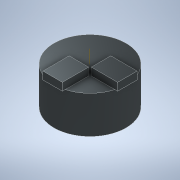
# Autodesk Inventor part: top tvc
Saved by Autodesk Inventor 2021 (Build 250183000, 183)
## iProperties
Created: 2021-07-19
Part Number: top tvc
Material: Iron, Cast
Document SubType Name: Modeling
Designer: samlo
Density: 7.15 g/cm^3
Appearance: Iron Gray
Author: samlo
Autodesk Inventor part; units mm, degrees
ref_plane "YZ Plane" through (0, 0, 0) normal (1, 0, 0) x (0, 1, 0)
ref_plane "XZ Plane" through (0, 0, 0) normal (0, 1, 0) x (-1, 0, 0)
ref_plane "XY Plane" through (0, 0, 0) normal (0, 0, 1) x (1, 0, 0)
sketch "Sketch1" plane through (0, 0, 0) normal (0, 0, 1) x (1, 0, 0)
  line L0 (22.1323, 8.4392) -> (22.1323, 23)
  line L1 (22.1323, 23) -> (0, 23)
  line L2 (0, 23) -> (0, 20)
  line L3 (0, -4.8284) -> (0, 28.9706) projected
  arc A0 (20, 0) -> (0, 20) centre (0, 0) ccw
  line L4 (22.1323, 8.4392) -> (22.1323, 0)
  line L5 (22.1323, 0) -> (20, 0)
  dimension "d4" = 40
  dimension "d5" = 23
  dimension "d6" = 3
  constraints: 10 end point, 3 perpendicular, 2 point on circle, 1 centre point, 1 coincident, 1 point on line, 1 vertical
  measures "d4" diameter of A0
  measures "d5" distance of L4.end L0.end
  measures "d6" distance of L2.end L1.end
revolve "Revolution1" add sketch "Sketch1" angle 360 about axis through (0, -10, 0) along (0, 1, 0)
sketch "Sketch2" plane through (0, 23, 0) normal (0, 1, 0) x (1, 0, 0)
  line L0 (-6, -6.8) -> (6, -6.8)
  line L1 (6, -6.8) -> (6, -23)
  line L2 (6, -23) -> (-6, -23)
  line L3 (-6, -23) -> (-6, -6.8)
  line L4 (0, 0) -> (30.3115, 0) construction
  dimension "d7" = 16.2
  dimension "d8" = 12
  dimension "d9" = 6
  dimension "d10" = 23
  constraints: 10 end point, 2 horizontal, 2 parallel, 1 perpendicular
  measures "d7" distance of L0.end L1.end
  measures "d8" distance of L1.end L2.end
  measures "d9" horizontal distance of L0.end L4.start
  measures "d10" distance from line of L2 L4.start
extrude "Extrusion1" add sketch "Sketch2" along normal blind 4.72
pattern_circular "Circular Pattern1" count 2 over 90 about axis through (0, -10, 0) along (0, 1, 0) of "Extrusion1"
body "Solid1"
